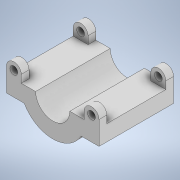
# Autodesk Inventor part: Relaxation chamber outer holder
Saved by Autodesk Inventor 2022 (Build 260153000, 153)
## iProperties
Created: 2021-11-15
Part Number: Relaxation chamber outer holder
Material: Generic
Document SubType Name: Modeling
Designer: Emazuddin Alif
Density: 1 g/cm^3
Appearance: Default
Author: Emazuddin Alif
Autodesk Inventor part; units mm, degrees
ref_plane "YZ Plane" through (0, 0, 0) normal (1, 0, 0) x (0, 1, 0)
ref_plane "XZ Plane" through (0, 0, 0) normal (0, 1, 0) x (-1, 0, 0)
ref_plane "XY Plane" through (0, 0, 0) normal (0, 0, 1) x (1, 0, 0)
sketch "Sketch1" plane through (0, 0, 0) normal (0, 0, 1) x (1, 0, 0)
  arc A0 (-13.9696, -0.1018) -> (13.9696, -0.1018) centre (0, 0) ccw
  line L0 (0, 64.951) -> (0, -100.8994)
  arc A1 (-23.2558, -13.0558) -> (23.2558, -13.0558) centre (0, 0) ccw
  line L1 (-23.2558, -13.0558) -> (-37.846, -13.0558)
  line L2 (37.846, -13.0558) -> (23.2558, -13.0558)
  arc A2 (-25.6593, 6.2482) -> (-37.846, 5.9942) centre (-31.75, 5.9942) ccw
  line L3 (-37.846, -0.3558) -> (-37.846, 5.9942)
  line L4 (-25.6593, -0.1018) -> (-25.6593, 6.2482)
  arc A3 (37.846, 5.9942) -> (25.6593, 6.2482) centre (31.75, 5.9942) ccw
  line L5 (37.846, -0.3558) -> (37.846, 5.9942)
  line L6 (25.6593, -0.1018) -> (25.6593, 6.2482)
  line L7 (-25.6593, -0.1018) -> (-13.9696, -0.1018)
  line L8 (13.9696, -0.1018) -> (25.6593, -0.1018)
  circle A4 centre (-31.75, 5.9942) radius 3.175
  circle A5 centre (31.75, 5.9942) radius 3.175
  line L9 (-37.846, -0.3558) -> (-37.846, -13.0558)
  line L10 (37.846, -0.3558) -> (37.846, -13.0558)
  dimension "d0" = 27.94
  dimension "d4" = 12.7
  dimension "d5" = 12.192
  dimension "d6" = 63.5
  dimension "d7" = 6.35
  dimension "d8" = 6.35
  dimension "d13" = 12.7
  dimension "d14" = 6.35
  dimension "d29" = 14.5902
  dimension "d31" = 14.5902
  dimension "d32" = 6.35
  constraints: 22 end point, 8 point on circle, 6 centre point, 5 symmetric about line, 4 coincident, 4 parallel, 3 vertical, 2 horizontal, 2 perpendicular, 2 tangent, 1 point on line, 1 other
  measures "d0" diameter of A0
  measures "d4" radial gap between concentric circles of A1 A0
  measures "d5" diameter of A2
  measures "d6" diameter of A2.centre L0
  measures "d7" diameter of A4
  measures "d8" diameter of A5
  measures "d13" distance of L3.start L1.end
  measures "d14" distance of L3.start L3.end
  measures "d29" distance of L1.start L1.end
  measures "d31" distance of L2.start L2.end
  measures "d32" distance of L4.start L4.end
extrude "Extrusion1" add sketch "Sketch1" along normal mid plane 60.96
sketch "Sketch3" plane through (-25.6593, -0.1018, 30.48) normal (1, 0, 0) x (0, 0, -1)
  line L0 (60.96, 0) -> (0, 0) projected
  line L1 (60.96, 12.192) -> (0, 12.192) projected
  line L2 (6.35, 0) -> (54.61, 0)
  line L3 (54.61, 0) -> (54.61, 12.192)
  line L4 (54.61, 12.192) -> (6.35, 12.192)
  line L5 (6.35, 12.192) -> (6.35, 0)
  line L6 (0, 12.192) -> (0, 6.096) projected
  line L7 (60.96, 6.35) -> (60.96, 12.192) projected
  point P0 (30.48, 0.1018)
  point P1 (6.35, 12.192)
  dimension "d23" = 6.35
  dimension "d24" = 6.35
  constraints: 8 end point, 2 parallel, 1 horizontal, 1 perpendicular, 1 point on line, 2 other
  measures "d23" distance between parallel lines of L6 L5
  measures "d24" distance between parallel lines of L7 L3
extrude "Extrusion3" cut sketch "Sketch3" along normal mid plane 152.4
body "Solid1"
